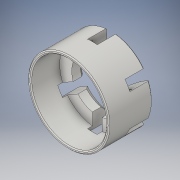
# Autodesk Inventor part: isolador v3_branco
Saved by Autodesk Inventor 2016 (Build 200138000, 138)
## iProperties
Created: 2016-08-17
Part Number: isolador v3_branco
Material: PPS Plastic
Document SubType Name: Modeling
Designer: fernando.santanna
Density: 1.637 g/cm^3
Appearance: Smooth - White
Author: fernando.santanna
Autodesk Inventor part; units mm, degrees
ref_plane "YZ Plane" through (0, 0, 0) normal (1, 0, 0) x (0, 1, 0)
ref_plane "Work Plane1" through (0, -11.700002, -0.000399) normal (0, 0, 1) x (1, 0, 0)
sketch "Sketch1" plane through (0, -11.700002, -0.000399) normal (0, 0, 1) x (1, 0, 0)
  circle A0 centre (-5.715, -3.175) radius 2.5781
  circle A1 centre (-5.715, -3.175) radius 3.95
  spline S0 degree 3 poles (-7.718488, -5.621666) (-7.626067, -5.697347) (-7.529433, -5.767729) (-7.328888, -5.897079) (-7.225154, -5.955968) (-6.904676, -6.11467) (-6.679725, -6.195976) (-6.29325, -6.288038) (-6.136162, -6.313152) (-5.773362, -6.343413) (-5.567695, -6.340525) (-5.161001, -6.295073) (-4.960904, -6.252841) (-4.571981, -6.130526) (-4.384045, -6.050793) (-4.024539, -5.85543) (-3.853983, -5.739953) (-3.537723, -5.477567) (-3.392764, -5.331287) (-3.134519, -5.014202) (-3.021545, -4.844386) (-2.832196, -4.489895) (-2.755396, -4.306482) (-2.665822, -4.019461) (-2.640108, -3.920413) (-2.578135, -3.623103) (-2.555967, -3.422435) (-2.550056, -3.01639) (-2.56695, -2.811947) (-2.640115, -2.408606) (-2.69633, -2.210683) (-2.845914, -1.829576) (-2.938729, -1.647211) (-3.15794, -1.303356) (-3.283738, -1.142619) (-3.56572, -0.846281) (-3.72149, -0.711617) (-4.056996, -0.474372) (-4.235943, -0.372366) (-4.609282, -0.205329) (-4.802638, -0.140341) (-5.197187, -0.048882) (-5.397382, -0.022245) (-5.700942, -0.011078) (-5.803262, -0.012278) (-6.106285, -0.030551) (-6.305611, -0.061827) (-6.698893, -0.162692) (-6.891773, -0.232679) (-7.261762, -0.409175) (-7.437951, -0.515358) (-7.766334, -0.759671) (-7.917889, -0.897048) (-8.192128, -1.198778) (-8.31423, -1.362371) (-8.526203, -1.712299) (-8.615276, -1.89799) (-8.756137, -2.284022) (-8.80759, -2.483445) (-8.870772, -2.8875) (-8.88273, -3.091119) (-8.867419, -3.496111) (-8.840513, -3.696559) (-8.771473, -3.992664) (-8.743435, -4.091069) (-8.646239, -4.378515) (-8.563762, -4.562504) (-8.363206, -4.915423) (-8.244992, -5.083194) (-7.977515, -5.393844) (-7.828821, -5.535933) (-7.506948, -5.788556) (-7.334669, -5.898678) (-6.971577, -6.084062) (-6.781641, -6.158942) (-6.388272, -6.271623) (-6.185671, -6.308822) (-5.776189, -6.343375) (-5.570281, -6.34066) (-5.163855, -6.295543) (-4.964254, -6.253624) (-4.577225, -6.132439) (-4.390613, -6.053711) (-4.12281, -5.909141) (-4.035235, -5.856229) (-3.783561, -5.686991) (-3.62782, -5.559163) (-3.340041, -5.273012) (-3.209183, -5.114837) (-2.979716, -4.775138) (-2.881702, -4.594382) (-2.722553, -4.217582) (-2.66157, -4.022516) (-2.578051, -3.623544) (-2.555675, -3.420579) (-2.550255, -3.01136) (-2.567577, -2.806066) (-2.64179, -2.401883) (-2.69848, -2.203949) (-2.848734, -1.823681) (-2.941595, -1.642106) (-3.160315, -1.300253) (-3.285489, -1.140653) (-3.495571, -0.920065) (-3.56964, -0.849483) (-3.80518, -0.64588) (-3.976533, -0.525172) (-4.340546, -0.31935) (-4.532312, -0.234743) (-4.828198, -0.137867) (-4.926861, -0.110782) (-5.224181, -0.044474) (-5.425472, -0.019486) (-5.831158, -0.008291) (-6.034616, -0.022321) (-6.437917, -0.089595) (-6.63675, -0.143052) (-7.02135, -0.287815) (-7.206193, -0.378801) (-7.554055, -0.594395) (-7.71644, -0.718197) (-8.01526, -0.995431) (-8.150974, -1.148242) (-8.39181, -1.478855) (-8.496171, -1.656019) (-8.668967, -2.027758) (-8.737051, -2.22143) (-8.833902, -2.615534) (-8.863153, -2.814881) (-8.878435, -3.117777) (-8.878631, -3.220094) (-8.864461, -3.524101) (-8.835725, -3.724597) (-8.740054, -4.118714) (-8.673079, -4.311359) (-8.502231, -4.682877) (-8.398412, -4.860718) (-8.157715, -5.19379) (-8.0214, -5.348221) (-7.722064, -5.627208) (-7.559989, -5.751363) (-7.213964, -5.966928) (-7.030792, -6.057784) (-6.648396, -6.203368) (-6.449993, -6.257535) (-6.045919, -6.326596) (-5.841217, -6.341407) (-5.435419, -6.331334) (-5.235244, -6.307163) (-4.938832, -6.242273) (-4.840057, -6.215571) (-4.550733, -6.122091) (-4.365096, -6.041813) (-4.010164, -5.846158) (-3.841851, -5.730947) (-3.528192, -5.468519) (-3.383831, -5.321627) (-3.125656, -5.001924) (-3.012456, -4.829875) (-2.821878, -4.46785) (-2.744639, -4.278891) (-2.627459, -3.888358) (-2.587868, -3.687675) (-2.547799, -3.280343) (-2.547638, -3.074634) (-2.587127, -2.666613) (-2.626585, -2.465255) (-2.74289, -2.076261) (-2.818841, -1.889338) (-2.959389, -1.620262) (-3.011106, -1.531967) (-3.177161, -1.277602) (-3.303189, -1.119784) (-3.584953, -0.828842) (-3.740314, -0.69666) (-4.0759, -0.462857) (-4.255556, -0.362103) (-4.631804, -0.196909) (-4.827495, -0.13285) (-5.226785, -0.043985) (-5.429368, -0.019049) (-5.837015, -0.008467) (-6.041129, -0.022944) (-6.444806, -0.091227) (-6.643381, -0.145085) (-7.026715, -0.290311) (-7.21061, -0.381225) (-7.555498, -0.595605) (-7.71602, -0.718044) (-7.938835, -0.92441) (-8.010452, -0.997502) (-8.210288, -1.222288) (-8.327913, -1.38273) (-8.534084, -1.727825) (-8.621343, -1.912179) (-8.75989, -2.296937) (-8.810494, -2.496566) (-8.87226, -2.902834) (-8.883271, -3.108507) (-8.865314, -3.517266) (-8.836738, -3.719404) (-8.741024, -4.115716) (-8.674043, -4.308948) (-8.503301, -4.680864) (-8.399737, -4.858578) (-8.186769, -5.153819) (-8.084274, -5.275455) (-7.806175, -5.559107) (-7.620559, -5.70992) (-7.319392, -5.902686) (-7.215467, -5.961206) (-7.00127, -6.066352) (-6.891157, -6.112867) (-6.778678, -6.153042) knots 0 0 0 0 0.03585853 0.03585853 0.07163771 0.07163771 0.14321275 0.14321275 0.19089992 0.19089992 0.25249885 0.25249885 0.31374538 0.31374538 0.37488634 0.37488634 0.43657051 0.43657051 0.4982446 0.4982446 0.5593293 0.5593293 0.61888803 0.61888803 0.64958873 0.64958873 0.71005601 0.71005601 0.77149243 0.77149243 0.833111 0.833111 0.89439427 0.89439427 0.95552421 0.95552421 1.0171905 1.0171905 1.07887685 1.07887685 1.13996876 1.13996876 1.20045734 1.20045734 1.2311569 1.2311569 1.29158774 1.29158774 1.35303824 1.35303824 1.41464547 1.41464547 1.47590675 1.47590675 1.53704433 1.53704433 1.59872305 1.59872305 1.66040252 1.66040252 1.72149045 1.72149045 1.78206506 1.78206506 1.81276347 1.81276347 1.87315422 1.87315422 1.93461994 1.93461994 1.99621436 1.99621436 2.05745112 2.05745112 2.11859734 2.11859734 2.18028788 2.18028788 2.2419592 2.2419592 2.30304327 2.30304327 2.36370568 2.36370568 2.39440299 2.39440299 2.45475045 2.45475045 2.51623227 2.51623227 2.57781256 2.57781256 2.63902246 2.63902246 2.70017828 2.70017828 2.76187962 2.76187962 2.82354151 2.82354151 2.88462197 2.88462197 2.94537197 2.94537197 2.97606827 2.97606827 3.0388358 3.0388358 3.10160331 3.10160331 3.13229923 3.13229923 3.19305035 3.19305035 3.25413064 3.25413064 3.31579297 3.31579297 3.37749363 3.37749363 3.43864992 3.43864992 3.49985968 3.49985968 3.56143896 3.56143896 3.62292161 3.62292161 3.68326811 3.68326811 3.71396503 3.71396503 3.77462865 3.77462865 3.83571249 3.83571249 3.89738427 3.89738427 3.95907416 3.95907416 4.0202208 4.0202208 4.08145745 4.08145745 4.14305085 4.14305085 4.20451737 4.20451737 4.2649072 4.2649072 4.29560521 4.29560521 4.35618108 4.35618108 4.41726876 4.41726876 4.4789487 4.4789487 4.54062677 4.54062677 4.60176474 4.60176474 4.66302595 4.66302595 4.72463215 4.72463215 4.78608343 4.78608343 4.8465134 4.8465134 4.87721255 4.87721255 4.9377024 4.9377024 4.99879402 4.99879402 5.06048085 5.06048085 5.12214651 5.12214651 5.1832768 5.1832768 5.24456003 5.24456003 5.30617758 5.30617758 5.36761474 5.36761474 5.42808123 5.42808123 5.45878151 5.45878151 5.51836937 5.51836937 5.57945414 5.57945414 5.64112932 5.64112932 5.70281193 5.70281193 5.76395262 5.76395262 5.82520099 5.82520099 5.8867999 5.8867999 5.9344807 5.9344807 6.00604561 6.00604561 6.04182032 6.04182032 6.07767461 6.07767461 6.07767461 6.07767461
  circle A2 centre (-5.715, -3.175) radius 2.5781
  circle A3 centre (-5.715, -3.175) radius 3.95
  circle A4 centre (-5.715, -3.175) radius 3.1623
  ellipse E0 centre (-5.715, -3.174686) end of major axis (-9.965, -3.174686) minor radius 4.25 (-3.669685, -6.900164) -> (-7.760315, -6.900164) ccw
  circle A5 centre (-5.715, -3.174686) radius 4.225
  circle A6 centre (-5.715, -3.174686) radius 2.65
  point P0 (0, 11.700002)
  dimension "d2" = 8.45
  dimension "d22" = 5.3
  dimension "d29" = 7.9
  constraints: 6 centre point, 5 coincident, 2 concentric, 1 other
  measures "d2" diameter of A5
  measures "d22" diameter of A6
  measures "d29" diameter of A1
sketch "Sketch1 outline for Extrusion1" plane through (0, -11.700002, -0.000399) normal (0, 0, 1) x (1, 0, 0)
  circle A0 centre (-5.715, -3.174686) radius 4.225
  circle A1 centre (-5.715, -3.174686) radius 2.65
extrude "Extrusion1" add sketch "Sketch1 outline for Extrusion1" along normal blind 1.5
sketch "Sketch2" plane through (-5.715, -14.874688, 1.499601) normal (0, 0, 1) x (1, 0, 0)
  circle A0 centre (0, -0.000314) radius 3.9
  circle A1 centre (0, 0) radius 4.225
  point P0 (5.715, 14.874688)
  dimension "d31" = 7.8
  constraints: 1 centre point
  measures "d31" diameter of A0
ref_plane "Work Plane2" through (-10.95, -21.800251, 4.174384) normal (0, -0.0000341, 1) x (1, 0, 0)
extrude "Extrusion2" add sketch "Sketch2" along normal blind 3
chamfer "Chamfer1" distance 0.1 angle 45 3 edges at (-9.94, -14.8747, -0.0004) (-9.94, -14.8747, 4.4996) (-9.615, -14.875, 4.4996)
sketch "Sketch3" plane through (-5.715, -14.874688, -0.000399) normal (0, 0, -1) x (-1, 0, 0)
  circle A0 centre (0, 0) radius 4.225
  circle A1 centre (0, -0.000314) radius 2.5781
  line L0 (-0.5, 4.527652) -> (0.5, 4.527652)
  line L1 (0.5, 4.527652) -> (0.5, 2.05543)
  line L2 (0.5, 2.05543) -> (-0.5, 2.05543)
  line L3 (-0.5, 2.05543) -> (-0.5, 4.527652)
  point P0 (-5.715, 14.874688)
  dimension "d13" = 1
  dimension "d14" = 0.5
  dimension "d15" = 2.47222
  dimension "d16" = 2.05574
  constraints: 8 end point, 2 parallel, 1 horizontal, 1 perpendicular
  measures "d13" distance of L0.start L0.end
  measures "d14" distance from line of A1.centre L1
  measures "d15" distance of L0.end L1.end
  measures "d16" distance from line of A1.centre L2
extrude "Extrusion3" cut sketch "Sketch3" against normal blind 2 contours L1 A1 L3 A0 | A0 L3 L0 L1 | L1 L2 L3 A1 picked at (0.389204, 3.098826) picked at (0.05587, 2.227731)
chamfer "Chamfer3" distance 0.6 angle 45 1 edges at (-5.715, -17.5247, -0.0004)
pattern_circular "Circular Pattern2" count 6 over 360 about axis through (-5.715, -14.874688, 0.299601) along (0, 0, -1) of "Extrusion3"
equation "\"d14\" = 0.5 * d13"
body "Solid1"
